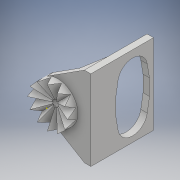
# Autodesk Inventor part: drzak
Saved by Autodesk Inventor 2018 (Build 220112000, 112)
## iProperties
Created: 2017-05-04
Part Number: drzak
Material: Všeobecné
Document SubType Name: Modeling
Designer: tonarr
Density: 1 g/cm^3
Appearance: Výchozí
Author: tonarr
Autodesk Inventor part; units mm, degrees
ref_plane "YZ Plane" through (0, 0, 0) normal (1, 0, 0) x (0, 1, 0)
ref_plane "XZ Plane" through (0, 0, 0) normal (0, 1, 0) x (-1, 0, 0)
sketch "Náčrt1" plane through (0, 0, 0) normal (0, 1, 0) x (-1, 0, 0)
  circle A0 centre (0, 0) radius 2
  circle A1 centre (0, 0) radius 12.5
  line L0 (6.7396, 10.5275) -> (-16.566, 25.4475)
  line L1 (-16.566, 25.4475) -> (-16.566, -24.5525)
  line L2 (-16.566, -24.5525) -> (6.4433, -10.7114)
  line L3 (-16.566, 25.4475) -> (-20.566, 25.4475)
  line L4 (-20.566, 25.4475) -> (-20.566, -24.5525)
  line L5 (-20.566, -24.5525) -> (-16.566, -24.5525)
  line L6 (-16.566, -24.5525) -> (-16.566, 25.4475)
  dimension "d0" = 4
  dimension "d1" = 25
  dimension "d2" = 50
  dimension "d3" = 4
  constraints: 14 end point, 2 centre point, 2 coincident, 2 parallel, 2 point on circle, 2 tangent, 1 horizontal, 1 perpendicular
  measures "d0" diameter of A0
  measures "d1" diameter of A1
  measures "d2" distance of L0.end L1.end
  measures "d3" distance of L4.end L5.end
extrude "Vysunutí1" add sketch "Náčrt1" along normal blind 4
sketch "Náčrt2" plane through (0, 4, 0) normal (0, 1, 0) x (1, 0, 0)
  line L0 (20.566, 24.5525) -> (16.566, 24.5525) projected
  line L1 (20.566, -25.4475) -> (20.566, 24.5525) projected
  line L2 (16.566, 24.5525) -> (20.566, 24.5525)
  line L3 (20.566, 24.5525) -> (20.566, -25.4475)
  line L4 (20.566, -25.4475) -> (16.566, -25.4475)
  line L5 (16.566, -25.4475) -> (16.566, 24.5525)
  point P0 (0, 0)
  constraints: 8 end point, 2 parallel, 1 horizontal, 1 perpendicular
extrude "Vysunutí2" add sketch "Náčrt2" along normal blind 35
sketch "Náčrt3" plane through (20.566, 0, 25.4475) normal (1, 0, 0) x (0, 0, -1)
  circle A0 centre (13.6975, 26) radius 9.25
  circle A1 centre (37.1975, 26) radius 9.25
  line L0 (0, 39) -> (50, 39) projected
  line L1 (25.4475, 0) -> (25.4475, 39)
  line L2 (50, 39) -> (0, 39) projected
  line L3 (20.4475, 15.5) -> (30.4475, 15.5)
  line L4 (20.4475, 15.5) -> (12.1796, 16.8754)
  line L5 (30.4475, 15.5) -> (38.7155, 16.8754)
  line L6 (20.4475, 36.5) -> (30.4475, 36.5)
  line L7 (20.4475, 36.5) -> (12.1796, 35.1246)
  line L8 (30.4475, 36.5) -> (38.7155, 35.1246)
  dimension "d8" = 18.5
  dimension "d9" = 23.5
  dimension "d10" = 13
  dimension "d11" = 13
  dimension "d12" = 11.75
  dimension "d13" = 10
  dimension "d14" = 5
  dimension "d15" = 10.5
  dimension "d16" = 18.5
  dimension "d17" = 10
  dimension "d18" = 5
  dimension "d19" = 10.5
  constraints: 14 end point, 4 point on circle, 4 tangent, 2 centre point, 2 horizontal, 1 perpendicular, 1 point on line
  measures "d8" diameter of A0
  measures "d9" distance of A1.centre A0.centre
  measures "d10" distance from line of L0 A0.centre
  measures "d11" distance from line of L0 A1.centre
  measures "d12" distance from line of L1 A0.centre
  measures "d13" distance of L3.start L3.end
  measures "d14" distance from line of L1 L3.end
  measures "d15" distance from line of L3 A0.centre
  measures "d16" diameter of A1
  measures "d17" distance of L6.start L6.end
  measures "d18" distance from line of L1 L6.end
  measures "d19" distance from line of A0.centre L6
extrude "Vysunutí3" cut sketch "Náčrt3" against normal blind 35
sketch "Náčrt4" plane through (0, 0, 0) normal (0, -1, 0) x (1, 0, 0)
  circle A0 centre (0, 0) radius 2 projected
  circle A1 centre (0, 0) radius 12.5
  constraints: 1 centre point, 1 coincident
extrude "Vysunutí4" add sketch "Náčrt4" along normal blind 7
sketch "Náčrt5" plane through (0, 4, 0) normal (0, 1, 0) x (1, 0, 0)
  line L0 (16.566, 24.5525) -> (-6.4433, 10.7114) projected
  line L1 (9.566, 20.3417) -> (9.566, 15.3417)
  line L2 (-6.7396, -10.5275) -> (16.566, -25.4475) projected
  line L3 (9.566, -20.9662) -> (9.566, -15.9662)
  line L4 (9.566, -15.9662) -> (16.566, -20.4475)
  line L5 (16.566, -25.4475) -> (16.566, 24.5525) projected
  line L6 (9.566, 15.3417) -> (16.566, 19.5525)
  line L7 (16.566, 24.5525) -> (16.566, -25.4475) projected
  point P0 (0, 0)
  dimension "d24" = 5
  dimension "d25" = 5
  dimension "d30" = 7
  dimension "d31" = 7
  constraints: 8 end point, 4 parallel, 4 point on line, 2 vertical
  measures "d24" distance of L1.start L1.end
  measures "d25" distance of L3.start L3.end
  measures "d30" distance between parallel lines of L5 L1
  measures "d31" distance between parallel lines of L5 L3
extrude "Vysunutí5" add sketch "Náčrt5" along normal blind 10
chamfer "Zkosení1" distance 6.75 distance2 10 1 edges at (9.566, 14, 18.4662) measured on face at (11.8993, 14, 19.1266)
chamfer "Zkosení2" distance 6.75 distance2 10 1 edges at (9.566, 14, -17.8417) measured on face at (11.8993, 14, -18.4119)
ref_plane "Pracovní rovina1" through (0, 0, 0) normal (0.2588, 0, 0.9659) x (0, 1, 0)
sketch "Náčrt6" plane through (0, -7, 0) normal (0, -1, 0) x (1, 0, 0)
  point P0 (0, 0)
sketch "Náčrt7" plane through (0, 0, 0) normal (0.2588, 0, 0.9659) x (0, 1, 0)
  line L0 (-0.9378, 0) -> (-7, -3.5)
  line L1 (-7, -3.5) -> (-7, 3.5)
  line L2 (-7, 3.5) -> (-0.9378, 0)
  line L3 (-7, 12.5) -> (-7, -12.5) projected
  line L4 (0, 3.4515) -> (4, 3.4515) projected
  line L5 (0, 9.2347) -> (0, 3.4515) projected
  line L6 (0, 9.2347) -> (4, 9.2347) projected
  line L7 (4, 3.4515) -> (4, 9.2347) projected
  point P0 (0, 0)
  point P1 (-4.9793, 0)
  point P2 (-7, 0)
  point P3 (-7, 0)
  dimension "d39" = 7
  constraints: 6 end point, 2 midpoint, 1 coincident, 1 horizontal alignment, 1 vertical, 7 other
  measures "d39" distance of L0.end L1.end
extrude "Vysunutí6" cut sketch "Náčrt7" against normal blind 18.5 contours L0 L1 L2
pattern_circular "Kruhové pole1" count 12 over 360 about axis through (0, -10, 0) along (0, 1, 0) of "Vysunutí6"
